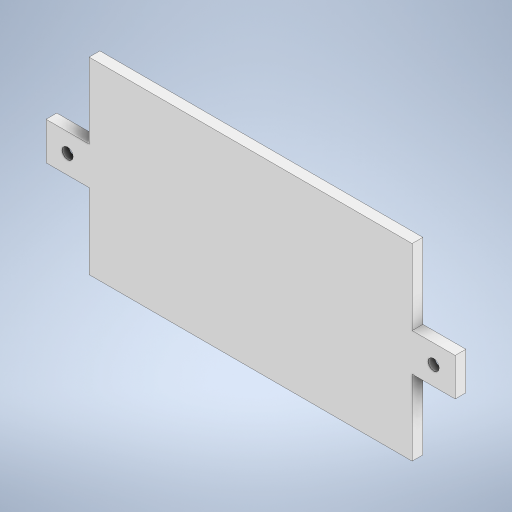
# Autodesk Inventor part: Coperchio
Saved by Autodesk Inventor 2023 (Build 270158000, 158)
## iProperties
Created: 2022-12-31
Part Number: Coperchio
Material: Plastica ABS
Document SubType Name: Modeling
Designer: Gabriele
Density: 1.06 g/cm^3
Appearance: Bianco
Author: Gabriele
Autodesk Inventor part; units mm, degrees
ref_plane "YZ Plane" through (0, 0, 0) normal (1, 0, 0) x (0, 1, 0)
ref_plane "XZ Plane" through (0, 0, 0) normal (0, 1, 0) x (-1, 0, 0)
ref_plane "XY Plane" through (0, 0, 0) normal (0, 0, 1) x (1, 0, 0)
sketch "Schizzo1" plane through (0, 0, 0) normal (0, 0, 1) x (1, 0, 0)
  line L0 (30.5, 18) -> (-30.5, 18)
  line L1 (-30.5, -18) -> (30.5, -18)
  line L2 (30.5, 18) -> (-30.5, -18) construction
  line L3 (-30.5, 18) -> (30.5, -18) construction
  line L4 (30.5, -4) -> (38.5, -4)
  line L5 (38.5, -4) -> (38.5, 4)
  line L6 (38.5, 4) -> (30.5, 4)
  line L7 (30.5, -18) -> (30.5, -4)
  line L8 (30.5, 4) -> (30.5, 18)
  line L9 (-30.5, -4) -> (-38.5, -4)
  line L10 (-38.5, -4) -> (-38.5, 4)
  line L11 (-38.5, 4) -> (-30.5, 4)
  line L12 (-30.5, 18) -> (-30.5, 4)
  line L13 (-30.5, -4) -> (-30.5, -18)
  line L14 (-30, 17.5) -> (30, 17.5)
  line L15 (30, 17.5) -> (30, 3.5)
  line L16 (30, 3.5) -> (38, 3.5)
  line L17 (38, 3.5) -> (38, -3.5)
  line L18 (38, -3.5) -> (30, -3.5)
  line L19 (30, -3.5) -> (30, -17.5)
  line L20 (30, -17.5) -> (-30, -17.5)
  line L21 (-30, -17.5) -> (-30, -3.5)
  line L22 (-30, -3.5) -> (-38, -3.5)
  line L23 (-38, -3.5) -> (-38, 3.5)
  line L24 (-38, 3.5) -> (-30, 3.5)
  line L25 (-30, 3.5) -> (-30, 17.5)
  point P0 (0, 0)
  dimension "d17" = 61
  dimension "d18" = 36
  dimension "d19" = 8
  dimension "d20" = 8
  dimension "d21" = 4
  dimension "d22" = 8
  dimension "d23" = 8
  dimension "d24" = 4
  dimension "d25" = 8
  dimension "d26" = 0.5
  constraints: 52 end point, 16 perpendicular, 10 parallel, 3 horizontal, 2 midpoint, 11 other
  measures "d17" distance of L1.start L1.end
  measures "d18" distance of L0.end L1.start
  measures "d19" distance of L5.end L6.end
  measures "d20" distance of L4.end L5.end
  measures "d21" distance from line of L6 point (0, 0)
  measures "d22" distance of L10.end L11.end
  measures "d23" distance of L9.end L10.end
  measures "d24" distance from line of point (0, 0) L11
  measures "d25" distance of L4.start L4.end
  measures "d26" distance between parallel lines of L0 L14
extrude "Estrusione1" add sketch "Schizzo1" along normal blind 2 contours L14 L15 L16 L17 L18 L19 L20 L21 L22 L23 L24 L25
sketch "Schizzo7" plane through (0, 0, 0) normal (0, 0, -1) x (-1, 0, 0)
  line L0 (-38, 3.5) -> (-30, 3.5) projected
  line L1 (30, 3.5) -> (38, 3.5) projected
  point P0 (0, 0)
  point P1 (34, 0)
  point P2 (-34, 0)
  dimension "d64" = 3.5
  dimension "d65" = 3.5
  dimension "d66" = 34
  dimension "d67" = 34
  measures "d64" distance from line of L0 point (-34, 0)
  measures "d65" distance from line of L1 point (34, 0)
  measures "d66" distance of point (0, 0) point (-34, 0)
  measures "d67" distance of point (0, 0) point (34, 0)
hole "Foro2" at (-34, 0, 0) at (34, 0, 0) direction (0, 0, 1) diameter 2.1 depth 8 countersink diameter 4.1 countersink angle 55
sketch "Schizzo8" plane through (0, 0, 0) normal (0, 0, -1) x (-1, 0, 0)
  line L0 (-6.2796, 12.7418) -> (-28.8271, 12.7418) construction
  line L1 (-28.8271, 12.7418) -> (-28.8271, 15.8738) construction
  line L2 (-28.8271, 15.8738) -> (-6.2796, 15.8738) construction
  line L3 (-6.2796, 15.8738) -> (-6.2796, 12.7418) construction
  line L4 (-7.2302, 15.387) -> (-7.2302, 12.217)
  line L5 (-7.2302, 12.217) -> (-8.2359, 12.217)
  spline S0 degree 2 poles (-8.2359, 12.217) (-8.6976, 12.217) (-9.2328, 12.6199) (-9.2328, 12.9404) knots 0 0 0 1 2 2 2
  spline S1 degree 2 poles (-9.2328, 12.9404) (-9.2328, 13.211) (-8.9299, 13.6079) (-8.6594, 13.6932) knots 0 0 0 1 2 2 2
  line L6 (-8.6594, 13.6932) -> (-8.6594, 13.702)
  spline S2 degree 2 poles (-8.6594, 13.702) (-8.9858, 13.7403) (-9.3769, 14.149) (-9.3769, 14.4754) knots 0 0 0 1 2 2 2
  spline S3 degree 2 poles (-9.3769, 14.4754) (-9.3769, 14.8842) (-8.7359, 15.387) (-8.2477, 15.387) knots 0 0 0 1 2 2 2
  line L7 (-8.2477, 15.387) -> (-7.2302, 15.387)
  line L8 (-7.7537, 13.9638) -> (-7.7537, 14.9665)
  line L9 (-7.7537, 14.9665) -> (-8.2036, 14.9665)
  spline S4 degree 2 poles (-8.2036, 14.9665) (-8.4977, 14.9665) (-8.8182, 14.696) (-8.8182, 14.4548) knots 0 0 0 1 2 2 2
  spline S5 degree 2 poles (-8.8182, 14.4548) (-8.8182, 13.9638) (-8.136, 13.9638) knots 0 0 0 1 1 1
  line L10 (-8.136, 13.9638) -> (-7.7537, 13.9638)
  line L11 (-7.7537, 12.6405) -> (-7.7537, 13.5403)
  line L12 (-7.7537, 13.5403) -> (-8.0948, 13.5403)
  spline S6 degree 2 poles (-8.0948, 13.5403) (-8.3683, 13.5403) (-8.68, 13.2815) (-8.68, 13.0463) knots 0 0 0 1 2 2 2
  spline S7 degree 2 poles (-8.68, 13.0463) (-8.68, 12.6405) (-8.136, 12.6405) knots 0 0 0 1 1 1
  line L13 (-8.136, 12.6405) -> (-7.7537, 12.6405)
  line L14 (-11.6471, 15.387) -> (-11.1472, 15.387)
  line L15 (-11.1472, 15.387) -> (-11.1472, 15.0342)
  line L16 (-11.1472, 15.0342) -> (-11.1383, 15.0342)
  spline S8 degree 2 poles (-11.1383, 15.0342) (-10.906, 15.44) (-10.4532, 15.44) knots 0 0 0 1 1 1
  spline S9 degree 2 poles (-10.4532, 15.44) (-10.1179, 15.44) (-9.7386, 15.0783) (-9.7386, 14.7783) knots 0 0 0 1 2 2 2
  spline S10 degree 2 poles (-9.7386, 14.7783) (-9.7386, 14.1373) (-10.4796, 14.0314) knots 0 0 0 1 1 1
  line L17 (-10.4796, 14.0314) -> (-11.1501, 13.9373)
  spline S11 degree 2 poles (-11.1501, 13.9373) (-11.1501, 13.4521) (-10.6914, 13.4521) knots 0 0 0 1 1 1
  spline S12 degree 2 poles (-10.6914, 13.4521) (-10.2856, 13.4521) (-9.9621, 13.7315) knots 0 0 0 1 1 1
  line L18 (-9.9621, 13.7315) -> (-9.9621, 13.2815)
  spline S13 degree 2 poles (-9.9621, 13.2815) (-10.3179, 13.0698) (-10.7884, 13.0698) knots 0 0 0 1 1 1
  spline S14 degree 2 poles (-10.7884, 13.0698) (-11.6471, 13.0698) (-11.6471, 13.9138) knots 0 0 0 1 1 1
  line L19 (-11.6471, 13.9138) -> (-11.6471, 15.387)
  line L20 (-11.1501, 14.2755) -> (-10.6737, 14.3431)
  spline S15 degree 2 poles (-10.6737, 14.3431) (-10.4532, 14.3696) (-10.2297, 14.5284) (-10.2297, 14.7254) knots 0 0 0 1 2 2 2
  spline S16 degree 2 poles (-10.2297, 14.7254) (-10.2297, 14.8695) (-10.4355, 15.0518) (-10.609, 15.0518) knots 0 0 0 1 2 2 2
  spline S17 degree 2 poles (-10.609, 15.0518) (-10.8443, 15.0518) (-11.1501, 14.7224) (-11.1501, 14.4725) knots 0 0 0 1 2 2 2
  line L21 (-11.1501, 14.4725) -> (-11.1501, 14.2755)
  spline S18 degree 2 poles (-13.4673, 15.3606) (-13.3144, 15.437) (-13.0703, 15.437) knots 0 0 0 1 1 1
  spline S19 degree 2 poles (-13.0703, 15.437) (-12.4116, 15.437) (-12.4116, 14.8048) knots 0 0 0 1 1 1
  line L22 (-12.4116, 14.8048) -> (-12.4116, 13.5256)
  line L23 (-12.4116, 13.5256) -> (-12.0323, 13.5256)
  line L24 (-12.0323, 13.5256) -> (-12.0323, 13.1227)
  line L25 (-12.0323, 13.1227) -> (-12.4116, 13.1227)
  line L26 (-12.4116, 13.1227) -> (-12.4116, 12.5993)
  line L27 (-12.4116, 12.5993) -> (-12.9233, 12.4523)
  line L28 (-12.9233, 12.4523) -> (-12.9233, 13.1227)
  line L29 (-12.9233, 13.1227) -> (-13.4673, 13.1227)
  line L30 (-13.4673, 13.1227) -> (-13.4673, 13.5256)
  line L31 (-13.4673, 13.5256) -> (-12.9233, 13.5256)
  line L32 (-12.9233, 13.5256) -> (-12.9233, 14.6577)
  spline S20 degree 2 poles (-12.9233, 14.6577) (-12.9233, 14.8577) (-13.0703, 15.0312) (-13.2409, 15.0312) knots 0 0 0 1 2 2 2
  spline S21 degree 2 poles (-13.2409, 15.0312) (-13.3703, 15.0312) (-13.4673, 14.9548) knots 0 0 0 1 1 1
  line L33 (-13.4673, 14.9548) -> (-13.4673, 15.3606)
  spline S22 degree 2 poles (-15.1023, 15.3606) (-14.9494, 15.437) (-14.7053, 15.437) knots 0 0 0 1 1 1
  spline S23 degree 2 poles (-14.7053, 15.437) (-14.0466, 15.437) (-14.0466, 14.8048) knots 0 0 0 1 1 1
  line L34 (-14.0466, 14.8048) -> (-14.0466, 13.5256)
  line L35 (-14.0466, 13.5256) -> (-13.6673, 13.5256)
  line L36 (-13.6673, 13.5256) -> (-13.6673, 13.1227)
  line L37 (-13.6673, 13.1227) -> (-14.0466, 13.1227)
  line L38 (-14.0466, 13.1227) -> (-14.0466, 12.5993)
  line L39 (-14.0466, 12.5993) -> (-14.5583, 12.4523)
  line L40 (-14.5583, 12.4523) -> (-14.5583, 13.1227)
  line L41 (-14.5583, 13.1227) -> (-15.1023, 13.1227)
  line L42 (-15.1023, 13.1227) -> (-15.1023, 13.5256)
  line L43 (-15.1023, 13.5256) -> (-14.5583, 13.5256)
  line L44 (-14.5583, 13.5256) -> (-14.5583, 14.6577)
  spline S24 degree 2 poles (-14.5583, 14.6577) (-14.5583, 14.8577) (-14.7053, 15.0312) (-14.8759, 15.0312) knots 0 0 0 1 2 2 2
  spline S25 degree 2 poles (-14.8759, 15.0312) (-15.0053, 15.0312) (-15.1023, 14.9548) knots 0 0 0 1 1 1
  line L45 (-15.1023, 14.9548) -> (-15.1023, 15.3606)
  line L46 (-17.4578, 14.3931) -> (-15.9169, 14.3931)
  spline S26 degree 2 poles (-15.9169, 14.3931) (-15.9257, 14.7077) (-16.2933, 15.0489) (-16.6167, 15.0489) knots 0 0 0 1 2 2 2
  spline S27 degree 2 poles (-16.6167, 15.0489) (-16.9784, 15.0489) (-17.2813, 14.8312) knots 0 0 0 1 1 1
  line L47 (-17.2813, 14.8312) -> (-17.2813, 15.2459)
  spline S28 degree 2 poles (-17.2813, 15.2459) (-16.9726, 15.44) (-16.4638, 15.44) knots 0 0 0 1 1 1
  spline S29 degree 2 poles (-16.4638, 15.44) (-15.9639, 15.44) (-15.3964, 14.8224) (-15.3964, 14.2637) knots 0 0 0 1 2 2 2
  spline S30 degree 2 poles (-15.3964, 14.2637) (-15.3964, 13.7344) (-16.0227, 13.0698) (-16.4874, 13.0698) knots 0 0 0 1 2 2 2
  spline S31 degree 2 poles (-16.4874, 13.0698) (-16.952, 13.0698) (-17.4578, 13.6668) (-17.4578, 14.1961) knots 0 0 0 1 2 2 2
  line L48 (-17.4578, 14.1961) -> (-17.4578, 14.3931)
  spline S32 degree 2 poles (-16.9637, 14.0314) (-16.9608, 13.755) (-16.705, 13.4492) (-16.4785, 13.4492) knots 0 0 0 1 2 2 2
  spline S33 degree 2 poles (-16.4785, 13.4492) (-16.258, 13.4492) (-15.9522, 13.7697) (-15.9169, 14.0314) knots 0 0 0 1 2 2 2
  line L49 (-15.9169, 14.0314) -> (-16.9637, 14.0314)
  spline S34 degree 2 poles (-19.2604, 13.6109) (-19.1692, 13.5374) (-18.9928, 13.5374) knots 0 0 0 1 1 1
  spline S35 degree 2 poles (-18.9928, 13.5374) (-18.7663, 13.5374) (-18.4605, 13.9491) (-18.4605, 14.3019) knots 0 0 0 1 2 2 2
  line L50 (-18.4605, 14.3019) -> (-18.4605, 15.387)
  line L51 (-18.4605, 15.387) -> (-17.9488, 15.387)
  line L52 (-17.9488, 15.387) -> (-17.9488, 13.1227)
  line L53 (-17.9488, 13.1227) -> (-18.4605, 13.1227)
  line L54 (-18.4605, 13.1227) -> (-18.4605, 13.5874)
  line L55 (-18.4605, 13.5874) -> (-18.4693, 13.5874)
  spline S36 degree 2 poles (-18.4693, 13.5874) (-18.5458, 13.3492) (-18.8575, 13.0816) (-19.0486, 13.0816) knots 0 0 0 1 2 2 2
  spline S37 degree 2 poles (-19.0486, 13.0816) (-19.1869, 13.0816) (-19.2604, 13.1227) knots 0 0 0 1 1 1
  line L56 (-19.2604, 13.1227) -> (-19.2604, 13.6109)
  line L57 (-21.5864, 13.1227) -> (-20.5631, 15.7487)
  spline S38 degree 2 poles (-20.5631, 15.7487) (-20.2455, 16.4515) (-19.6691, 16.4515) knots 0 0 0 1 1 1
  spline S39 degree 2 poles (-19.6691, 16.4515) (-19.5074, 16.4515) (-19.4015, 16.4221) knots 0 0 0 1 1 1
  line L58 (-19.4015, 16.4221) -> (-19.4015, 15.9957)
  spline S40 degree 2 poles (-19.4015, 15.9957) (-19.5221, 16.0369) (-19.6221, 16.0369) knots 0 0 0 1 1 1
  spline S41 degree 2 poles (-19.6221, 16.0369) (-19.9102, 16.0369) (-20.0514, 15.7546) knots 0 0 0 1 1 1
  line L59 (-20.0514, 15.7546) -> (-20.2043, 15.3811)
  line L60 (-20.2043, 15.3811) -> (-19.3045, 13.1227)
  line L61 (-19.3045, 13.1227) -> (-19.872, 13.1227)
  line L62 (-19.872, 13.1227) -> (-20.4102, 14.7666)
  spline S42 degree 2 poles (-20.4102, 14.7666) (-20.419, 14.7989) (-20.4513, 14.9312) knots 0 0 0 1 1 1
  line L63 (-20.4513, 14.9312) -> (-20.4631, 14.9312)
  spline S43 degree 2 poles (-20.4631, 14.9312) (-20.4719, 14.8783) (-20.5013, 14.7695) knots 0 0 0 1 1 1
  line L64 (-20.5013, 14.7695) -> (-21.0689, 13.1227)
  line L65 (-21.0689, 13.1227) -> (-21.5864, 13.1227)
  spline S44 degree 2 poles (-25.1505, 13.6285) (-25.1505, 14.1049) (-24.9446, 14.7901) (-24.5859, 15.2341) (-24.1006, 15.4429) (-23.8213, 15.4429) knots 0 0 0 1 2 3 4 4 4
  spline S45 degree 2 poles (-23.8213, 15.4429) (-23.7331, 15.4429) (-23.5478, 15.4194) (-23.3831, 15.3841) (-23.2479, 15.3429) (-23.2038, 15.3223) knots 0 0 0 1 2 3 4 4 4
  line L66 (-23.2038, 15.3223) -> (-23.2038, 14.8607)
  spline S46 degree 2 poles (-23.2038, 14.8607) (-23.2508, 14.8901) (-23.3861, 14.9489) (-23.5478, 14.9959) (-23.7242, 15.0253) (-23.8036, 15.0253) knots 0 0 0 1 2 3 4 4 4
  spline S47 degree 2 poles (-23.8036, 15.0253) (-23.9918, 15.0253) (-24.3006, 14.8783) (-24.5153, 14.5931) (-24.6329, 14.1667) (-24.6329, 13.8844) knots 0 0 0 1 2 3 4 4 4
  line L67 (-24.6329, 13.8844) -> (-24.6241, 13.8844)
  spline S48 degree 2 poles (-24.6241, 13.8844) (-24.5859, 13.9549) (-24.4535, 14.0814) (-24.2859, 14.1755) (-24.0801, 14.2343) (-23.9654, 14.2343) knots 0 0 0 1 2 3 4 4 4
  spline S49 degree 2 poles (-23.9654, 14.2343) (-23.7654, 14.2343) (-23.4214, 14.0961) (-23.1714, 13.8373) (-23.0273, 13.4727) (-23.0273, 13.2462) knots 0 0 0 1 2 3 4 4 4
  spline S50 degree 2 poles (-23.0273, 13.2462) (-23.0273, 12.9992) (-23.1891, 12.5964) (-23.4772, 12.317) (-23.8654, 12.1641) (-24.0948, 12.1641) knots 0 0 0 1 2 3 4 4 4
  spline S51 degree 2 poles (-24.0948, 12.1641) (-24.3094, 12.1641) (-24.6917, 12.3258) (-24.9799, 12.6758) (-25.1505, 13.2345) (-25.1505, 13.6285) knots 0 0 0 1 2 3 4 4 4
  spline S52 degree 2 poles (-24.6153, 13.2904) (-24.6153, 13.1316) (-24.5359, 12.8728) (-24.3888, 12.6875) (-24.1859, 12.5846) (-24.0683, 12.5846) knots 0 0 0 1 2 3 4 4 4
  spline S53 degree 2 poles (-24.0683, 12.5846) (-23.9624, 12.5846) (-23.7684, 12.6699) (-23.6243, 12.8287) (-23.5419, 13.0551) (-23.5419, 13.1933) knots 0 0 0 1 2 3 4 4 4
  spline S54 degree 2 poles (-23.5419, 13.1933) (-23.5419, 13.3433) (-23.6243, 13.5727) (-23.7684, 13.7285) (-23.9742, 13.8108) (-24.0977, 13.8108) knots 0 0 0 1 2 3 4 4 4
  spline S55 degree 2 poles (-24.0977, 13.8108) (-24.2095, 13.8108) (-24.3977, 13.7285) (-24.5359, 13.5903) (-24.6153, 13.3992) (-24.6153, 13.2904) knots 0 0 0 1 2 3 4 4 4
  line L68 (-28.2381, 12.217) -> (-27.1001, 15.387)
  line L69 (-27.1001, 15.387) -> (-26.512, 15.387)
  line L70 (-26.512, 15.387) -> (-25.3945, 12.217)
  line L71 (-25.3945, 12.217) -> (-25.9679, 12.217)
  line L72 (-25.9679, 12.217) -> (-26.7502, 14.6225)
  spline S56 degree 2 poles (-26.7502, 14.6225) (-26.7884, 14.7371) (-26.809, 14.8901) knots 0 0 0 1 1 1
  line L73 (-26.809, 14.8901) -> (-26.8178, 14.8901)
  spline S57 degree 2 poles (-26.8178, 14.8901) (-26.8325, 14.7636) (-26.8825, 14.6166) knots 0 0 0 1 1 1
  line L74 (-26.8825, 14.6166) -> (-27.6823, 12.217)
  line L75 (-27.6823, 12.217) -> (-28.2381, 12.217)
  point P0 (0, 0)
  constraints: 2 other
extrude "Estrusione5" cut sketch "Schizzo8" against normal blind 1
